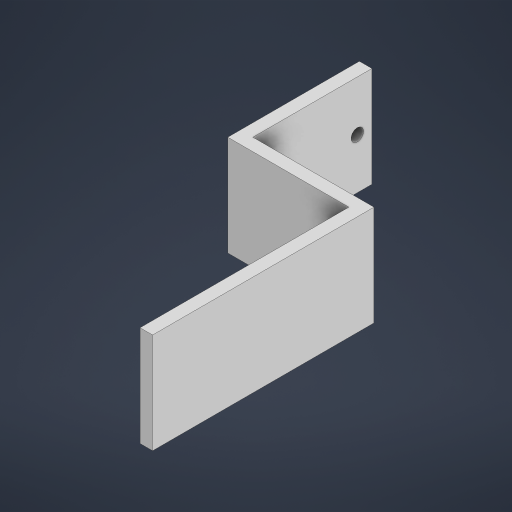
# Autodesk Inventor part: acople_2
Saved by Autodesk Inventor 2023.1 (Build 271208000, 208)
## iProperties
Created: 2022-10-23
Part Number: acople_2
Material: Generic
Document SubType Name: Modeling
Designer: amtat
Density: 1 g/cm^3
Appearance: Default
Author: amtat
Autodesk Inventor part; units mm, degrees
ref_plane "YZ Plane" through (0, 0, 0) normal (1, 0, 0) x (0, 1, 0)
ref_plane "XZ Plane" through (0, 0, 0) normal (0, 1, 0) x (-1, 0, 0)
ref_plane "XY Plane" through (0, 0, 0) normal (0, 0, 1) x (1, 0, 0)
sketch "Sketch1" plane through (0, 0, 0) normal (1, 0, 0) x (0, 1, 0)
  circle A0 centre (0, 0) radius 1.5
  circle A1 centre (0, -20) radius 1.5
  line L0 (0, 0) -> (12, 0)
  line L1 (12, 0) -> (12, -20)
  line L2 (0, 0) -> (-12, 0)
  line L3 (-12, 0) -> (-12, -20)
  arc A2 (0, -16.5) -> (0, -23.5) centre (0, -20) ccw
  line L4 (12, -20) -> (12, -23.5)
  line L5 (12, -23.5) -> (-12, -23.5)
  line L6 (-12, -23.5) -> (-12, -20)
  line L7 (0, 0) -> (0, -1.5)
  line L8 (0, -16.5) -> (0, -20)
  line L9 (12, 0) -> (12, 5)
  line L10 (12, 5) -> (-12, 5)
  line L11 (-12, 5) -> (-12, 0)
  dimension "d0" = 3
  dimension "d1" = 20
  dimension "d2" = 3
  dimension "d3" = 12
  dimension "d4" = 12
  dimension "d5" = 7
  dimension "d6" = 5
  constraints: 24 end point, 8 perpendicular, 4 vertical, 3 coincident, 2 centre point, 2 point on circle, 1 horizontal, 1 midpoint, 1 vertical alignment, 2 other
  measures "d1" distance of L0.start L8.end
  measures "d2" diameter of A1
  measures "d3" distance of L0.start L0.end
  measures "d4" distance of L0.start L2.end
  measures "d5" diameter of A2
  measures "d6" distance of L0.end L9.end
extrude "Extrusion1" add sketch "Sketch1" along normal blind 3 contours A0 L0 L1 L4 L5 L6 L3 L2 | A0 L2 L11 L10 L9 L0
sketch "Sketch2" plane through (0, 0, 0) normal (-1, 0, 0) x (0, 0, 1)
  line L0 (-23.5, 12) -> (5, 12) projected
  line L1 (-23.5, -12) -> (-23.5, 12) projected
  line L2 (5, -12) -> (-23.5, -12) projected
  line L3 (5, 12) -> (5, -12) projected
  circle A0 centre (-20, 0) radius 1.5 projected
  circle A1 centre (0, 0) radius 1.5 projected
  line L4 (5, 12) -> (5, -12) projected
  line L5 (5, -12) -> (8, -12)
  line L6 (8, -12) -> (8, 12)
  line L7 (-23.5, 12) -> (5, 12) projected
  line L8 (8, 12) -> (5, 12)
  dimension "d9" = 3
  constraints: 6 end point, 2 perpendicular, 1 horizontal
  measures "d9" distance of L2.start L5.end
extrude "Extrusion2" add sketch "Sketch2" against normal blind 32 contours L8 L6 L5 L3
sketch "Sketch3" plane through (0, -12, 8) normal (0, 0, 1) x (1, 0, 0)
  line L0 (0, 0) -> (0, 24) projected
  line L1 (0, 0) -> (32, 0) projected
  line L2 (32, 24) -> (32, 0) projected
  line L3 (0, 24) -> (32, 24) projected
  line L4 (32, 24) -> (32, 0) projected
  line L5 (32, 0) -> (29, 0)
  line L6 (0, 0) -> (32, 0) projected
  line L7 (29, 0) -> (29, 24)
  line L8 (0, 24) -> (32, 24) projected
  point P0 (0, 12)
  dimension "d12" = 3
  constraints: 4 end point, 2 point on line, 1 perpendicular
  measures "d12" distance of L1.end L5.end
extrude "Extrusion3" add sketch "Sketch3" along normal blind 50 contours L7 L3 L2 L1
body "Solid1"
